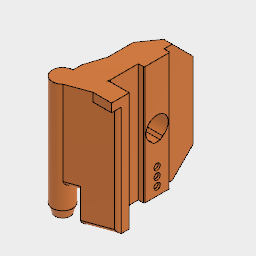
rambo_lid_upper_hinge v2 (Autodesk Fusion 360 design; units mm, degrees)
Autodesk Fusion 360 part; units mm, degrees
sketch "hinge_profile" plane through (0, 0, 0) normal (0, 0, 1) x (1, 0, 0)
  circle A0 centre (0, 0) radius 2.45
  line L0 (0, 4.5) -> (0, -2.45)
  line L1 (11.4, 4.5) -> (0, 4.5)
  line L2 (-0.2607, -2.4361) -> (11.4, 1.8081)
  line L3 (1.7335, -1.9763) -> (-0.0607, -2.6293) construction
  line L4 (11.4, 0.2) -> (6.9819, 0.2)
  line L5 (11.4, 0.2) -> (11.4, 4.5)
  line L6 (0, 4.5) -> (1.5, 9.25)
  arc A1 (4.8141, -0.589) -> (0.1101, 4.8487) centre (0, 0) ccw
  line L7 (6.5, 4.5) -> (6.5, 24.5)
  line L8 (6.5, 24.5) -> (1.5, 24.5)
  line L9 (1.5, 9.25) -> (1.5, 24.5)
  line L10 (7.9, 11.65) -> (7.9, 17.35)
  line L11 (7.9, 14.5) -> (6.5, 14.5) construction
  line L12 (6.5, 10.275) -> (6.725, 10.275)
  line L13 (6.5, 18.725) -> (6.725, 18.725)
  line L14 (7.7, 17.55) -> (6.5, 17.55)
  line L15 (7.7, 11.45) -> (6.5, 11.45)
  arc A2 (7.9, 17.35) -> (7.7, 17.55) centre (7.7, 17.35) ccw
  arc A3 (7.7, 11.45) -> (7.9, 11.65) centre (7.7, 11.65) ccw
  point P0 (7.9, 17.55)
  dimension "d2182" = 4.9
  dimension "d2227" = 0
  dimension "d2228" = 0
  dimension "d2229" = 0
  dimension "d2230" = 0
  dimension "d2241" = 0.25
  dimension "d61" = 2.4
  dimension "d123" = 5
  dimension "d124" = 4.3
  dimension "d126" = 20
  dimension "d127" = 20
  dimension "d128" = 4.9
  dimension "d132" = 10
  dimension "d133" = 1.4
  dimension "d141" = 5.25
  dimension "d142" = 4.5
  dimension "d165" = 1.5
  dimension "d198" = 0.2
  measures "d2182" diameter of A0
  measures "d2241" distance of L2 L3
  measures "d61" distance of A0 A1
  measures "d123" distance of L7.end L8.end
  measures "d124" distance of L1.start L4.start
  measures "d126" angle of L2 L4
  measures "d127" distance of L1.start L7.end
  measures "d128" distance of L1.start L7.start
  measures "d132" distance of L7.end L11.start
  measures "d133" distance of L7 P0
  measures "d141" distance of L6.end L11.end
  measures "d142" distance of A0.centre L1
  measures "d165" distance of A0.centre L8.end
  measures "d198" radius of A2
extrude "Extrude1" add sketch "hinge_profile" against normal blind 21 contours A0 L0 L2 | A0 L0 L2 | A0 L0 L2 | A0 L0 L1 L2 A1 | A0 L0 L2 | L1 L6 A1 | L1 L2 L5 A1 | L1 L6 A1 L7 L8 L9 | L7 L10 L14 L15 A2 A3
extrude "Extrude26" add sketch "hinge_profile" against normal blind 2 contours L2 L4 L5
extrude "Extrude2" add sketch "hinge_profile" against normal blind 7 from surface at -21 contours A0 L0 L2 | A0 L0 L2 | A0 L0 L2 | A0 L0 L2
extrude "Extrude21" add sketch "hinge_profile" against normal up to surface (7 mm away) from surface at -21 contours L1 L2 L5 A1 | L1 L6 A1 L7 L8 L9 | L7 L10 L14 L15 A2 A3
extrude "Extrude31" cut 1 faces at (9.7667, 4.5, -18.6667) along direction (0, -1, 0) blind 0.1
chamfer "Chamfer5" distance 0.65 distance2 2 1 edges at (-2.2842, 0.886, -28) measured on face at (-0.5987, 0.5555, -28)
sketch "frame_hole" plane through (1.5, 0, 0) normal (-1, 0, 0) x (0, -1, 0)
  line L0 (-9.25, 0) -> (-24.5, 0)
  line L1 (-24.5, 0) -> (-24.5, -28)
  line L2 (-24.5, -28) -> (-9.25, -28)
  line L3 (-9.25, -28) -> (-9.25, 0)
  line L4 (-24.5, 0) -> (-24.5, -28)
  line L5 (-24.5, -14) -> (-14.5, -14) construction
  circle A0 centre (-14.5, -14) radius 2.65
  circle A1 centre (-14.5, -14) radius 5.25
  line L6 (-24.5, -28) -> (-9.25, -28)
  line L7 (-19.75, -14) -> (-19.75, -28)
  line L8 (-9.25, 0) -> (-9.25, -28)
  line L9 (-15.825, -16.295) -> (-15.269, -16.851)
  line L10 (-15.269, -16.851) -> (-13.731, -16.851)
  line L11 (-13.731, -16.851) -> (-13.175, -16.295)
  line L12 (-14.5, -16.851) -> (-14.5, -14) construction
  dimension "d138" = 5.3
  dimension "d139" = 10.5
  dimension "d140" = 10
  dimension "d181" = 0.201
  dimension "d182" = 45
  dimension "d183" = 2.65
  measures "d138" diameter of A0
  measures "d139" diameter of A1
  measures "d140" distance of L5.start L5.end
  measures "d181" distance of A0 L10
  measures "d182" angle of L10 L11
  measures "d183" distance of L9.start L11.end
extrude "Extrude27" cut sketch "frame_hole" against normal blind 14 contours A0 | A0 L9 L10 L11
extrude "Extrude28" cut sketch "frame_hole" along normal blind 10 from surface at -1.5 contours A1 | L2 L3 A1 L6 L7 L8 | A0 L9 L10 L11
chamfer "Chamfer14" distance 5 angle 45 2 edges at (4, 24.5, -28) (4, 24.5, 0)
sketch "selective_infill" plane through (0, 0, -28) normal (0, 0, -1) x (1, 0, 0)
  circle A0 centre (0, 0) radius 2.45
  circle A1 centre (0, 0) radius 0.0505
  circle A2 centre (0, 0) radius 1.8
  dimension "d107" = 0.101
  measures "d107" diameter of A1
extrude "Extrude24" cut sketch "selective_infill" against normal up to surface (6 mm away) from surface at -1 contours A1
sketch "better_printed_angle" plane through (0, 0, 0) normal (0, 0, 1) x (-1, 0, 0)
  line L0 (-6.5, -19.5) -> (-1.5, -19.5)
  line L1 (-1.5, -19.5) -> (-1.5, -9.25)
  line L2 (-1.5, -9.25) -> (0, -4.5)
  line L3 (0, -4.5) -> (0, -2.45)
  arc A0 (0, -2.45) -> (-1.7656, 1.6986) centre (0, 0) ccw
  line L4 (-1.7656, 1.6986) -> (-6.9819, -0.2)
  line L5 (-6.9819, -0.2) -> (-11.4, -0.2)
  line L6 (-11.4, -0.2) -> (-11.4, -4.4)
  line L7 (-11.4, -4.4) -> (-6.5, -4.4)
  line L8 (-6.5, -4.4) -> (-6.5, -11.45)
  line L9 (-7.9, -11.65) -> (-7.9, -17.35)
  line L10 (-6.5, -4.4) -> (-6.5, -11.45)
  line L11 (-11.4, -4.4) -> (-6.5, -4.4)
  line L12 (-6.5, -4.85) -> (-6.3409, -4.2409)
  line L13 (-6.3409, -4.2409) -> (-6.95, -4.4)
  line L14 (-6.5, -4.4) -> (-6.3409, -4.2409) construction
  line L15 (-6.5, -11.45) -> (-7.7, -11.45)
  arc A1 (-7.7, -11.45) -> (-7.9, -11.65) centre (-7.7, -11.65) ccw
  arc A2 (-7.9, -17.35) -> (-7.7, -17.55) centre (-7.7, -17.35) ccw
  line L16 (-7.7, -17.55) -> (-6.5, -17.55)
  line L17 (-6.5, -17.55) -> (-6.5, -19.5)
  dimension "d192" = 135
  dimension "d193" = 0.45
  dimension "d194" = 0.45
  dimension "d195" = 0.225
  measures "d192" angle of L11 L14
  measures "d193" distance of L13.end L7.end
  measures "d194" distance of L12.start L7.end
  measures "d195" distance of L12.end L7.end
extrude "Extrude34" cut sketch "better_printed_angle" against normal blind 30 contours L7 L8 L10 L11 L12 L13
chamfer "Chamfer16" distance 3 angle 45 3 edges at (1.5, 22.125, -25.375) (1.5, 22, -2.5) (1.5, 24.5, -14)
fillet "Fillet4" radius 1 4 edges at (3.2899, -1.1438, -21) (11.4, 1.8081, -15) (8.1071, 0.6095, -28) (3.668, 3.173, -28)
sketch "mk_type" plane through (7.9, 0, 0) normal (1, 0, 0) x (0, 1, 0)
  line L0 (15.269, -16.851) -> (13.731, -16.851)
  line L1 (13.731, -16.851) -> (13.175, -16.295)
  arc A0 (15.825, -16.295) -> (13.175, -16.295) centre (14.5, -14) ccw
  line L2 (15.825, -16.295) -> (15.269, -16.851)
  line L3 (17.35, 0) -> (11.65, 0)
  line L4 (11.65, -28) -> (17.35, -28)
  line L5 (11.65, -28) -> (17.35, -28)
  line L6 (14.5, -28) -> (14.5, -22) construction
  circle A1 centre (14.5, -22) radius 0.75
  circle A2 centre (14.5, -24) radius 0.75
  circle A3 centre (14.5, -26) radius 0.75
  line L7 (11.65, 0) -> (11.65, -28)
  line L8 (17.35, -28) -> (17.35, 0)
  dimension "d184" = 1.5
  dimension "d185" = 1.5
  dimension "d186" = 1.5
  dimension "d187" = 2
  dimension "d188" = 2
  dimension "d189" = 2
  measures "d184" diameter of A1
  measures "d185" diameter of A2
  measures "d186" diameter of A3
  measures "d187" distance of L5 A3.centre
  measures "d188" distance of A2.centre A3.centre
  measures "d189" distance of L6.end A2.centre
extrude "Extrude33" cut sketch "mk_type" against normal blind 0.5 contours A1 | A2 | A3
equation "m5_hole_dia = 5.3 mm"
equation "m5_head_dia = 10.5 mm"
equation "d9 = 2.45 mm - 1.8 mm"
equation "layer_height = 0.2 mm"
equation "extrusion_width = 0.45 mm"
equation "num_perimeters = 3"
equation "perimeters_thickness = num_perimeters * extrusion_width - 0.1 mm"
equation "num_top_bottom = 5"
equation "top_bottom_thickness = num_top_bottom * layer_height"
equation "d112 = -top_bottom_thickness"
equation "d133 = rail_profile_height"
equation "d138 = m5_hole_dia"
equation "d139 = m5_head_dia"
equation "d141 = m5_head_dia / 2"
equation "rail_profile_width = 8.9 mm"
equation "rail_profile_height = 1.4 mm"
equation "d181 = layer_height + 0.001 mm"
equation "d183 = d138 / 2"
equation "d185 = d184"
equation "d186 = d184"
equation "d188 = d187"
equation "d189 = d188"
equation "d193 = extrusion_width"
equation "d194 = extrusion_width"
equation "d195 = extrusion_width / 2"
